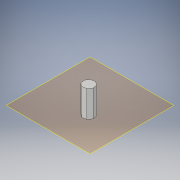
# Autodesk Inventor part: pin_oct_3mm
Saved by Autodesk Inventor 2019 (Build 230136000, 136)
## iProperties
Created: 2018-12-20
Part Number: pin_oct_3mm
Material: Generic
Document SubType Name: Modeling
Designer: assman
Density: 1 g/cm^3
Appearance: Default
Author: assman
## iProperties of the stored document pin_oct_3mm_3DPrint.ipt
Created: 2018-12-20
Part Number: pin_oct_3mm_3DPrint
Material: Generic
Document SubType Name: Modeling
Designer: assman
Density: 1 g/cm^3
Appearance: Default
Author: assman
Autodesk Inventor part; units mm, degrees
ref_plane "YZ Plane" through (0, 0, 0) normal (1, 0, 0) x (0, 1, 0)
ref_plane "XZ Plane" through (0, 0, 0) normal (0, 1, 0) x (-1, 0, 0)
ref_plane "XY Plane" through (0, 0, 0) normal (0, 0, 1) x (1, 0, 0)
ref_plane "Work Plane1" through (-10, 7, -20) normal (0, 1, 0) x (1, 0, 0)
sketch "Sketch3" plane through (-10, 7, -20) normal (0, 1, 0) x (1, 0, 0)
  circle A0 centre (1.9876, -2.3189) radius 1.5 construction
  line L0 (1.1839, -1.0524) -> (2.3148, -0.855)
  line L1 (2.3148, -0.855) -> (3.2541, -1.5151)
  line L2 (3.2541, -1.5151) -> (3.4515, -2.6461)
  line L3 (3.4515, -2.6461) -> (2.7914, -3.5854)
  line L4 (2.7914, -3.5854) -> (1.6605, -3.7828)
  line L5 (1.6605, -3.7828) -> (0.7212, -3.1227)
  line L6 (0.7212, -3.1227) -> (0.5238, -1.9917)
  line L7 (0.5238, -1.9917) -> (1.1839, -1.0524)
  point P0 (10, -20)
  constraints: 16 end point, 1 coincident, 19 other
extrude "Extrusion1" add sketch "Sketch3" along normal blind 7
body "Solid2"
body "Solid1"
